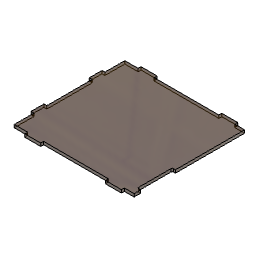
Deck Plate (Autodesk Fusion 360 design; units mm, degrees)
Autodesk Fusion 360 part; units mm, degrees
sketch "Sketch1" plane through (0, 0, 0) normal (0, 0, 1) x (1, 0, 0)
  line L0 (160, -90) -> (-160, -90)
  line L1 (-160, -90) -> (-160, 90)
  line L2 (-160, 90) -> (160, 90)
  line L3 (160, 90) -> (160, -90)
  line L4 (160, -90) -> (-160, 90) construction
  line L5 (-160, -90) -> (160, 90) construction
  line L6 (170, 85.5) -> (-180, 85.5) construction
  line L7 (-180, -85.5) -> (170, -85.5) construction
  line L8 (-155.5, 90) -> (-155.5, -90)
  line L9 (-160, 90) -> (-135, 90)
  line L10 (-135, 90) -> (-135, 85.5)
  line L11 (-135, 85.5) -> (-160, 85.5)
  line L12 (-160, 85.5) -> (-160, 90)
  line L13 (-160, -90) -> (-135, -90)
  line L14 (-135, -90) -> (-135, -85.5)
  line L15 (-135, -85.5) -> (-160, -85.5)
  line L16 (-160, -85.5) -> (-160, -90)
  line L17 (-110, -90) -> (-10, -90)
  line L18 (-10, -90) -> (-10, -85.5)
  line L19 (-10, -85.5) -> (-110, -85.5)
  line L20 (-110, -85.5) -> (-110, -90)
  line L21 (-10, -90) -> (15, -90)
  line L22 (15, -90) -> (15, -85.5)
  line L23 (15, -85.5) -> (-10, -85.5)
  line L24 (-10, -85.5) -> (-10, -90)
  line L25 (15, -90) -> (115, -90)
  line L26 (115, -85.5) -> (15, -85.5)
  line L27 (15, -85.5) -> (15, -90)
  line L28 (115, -90) -> (140, -90)
  line L29 (140, -85.5) -> (115, -85.5)
  line L30 (-135, 85.5) -> (-110, 85.5)
  line L31 (-110, 85.5) -> (-110, 90)
  line L32 (-110, 90) -> (-135, 90)
  line L33 (-135, 90) -> (-135, 85.5)
  line L34 (-110, 85.5) -> (-10, 85.5)
  line L35 (-10, 85.5) -> (-10, 90)
  line L36 (-10, 90) -> (-110, 90)
  line L37 (-110, 90) -> (-110, 85.5)
  line L38 (-10, 85.5) -> (15, 85.5)
  line L39 (15, 85.5) -> (15, 90)
  line L40 (15, 90) -> (-10, 90)
  line L41 (-10, 90) -> (-10, 85.5)
  line L42 (15, 85.5) -> (115, 85.5)
  line L43 (115, 90) -> (15, 90)
  line L44 (15, 90) -> (15, 85.5)
  line L45 (115, 85.5) -> (140, 85.5)
  line L46 (140, 90) -> (115, 90)
  line L47 (140, 85.5) -> (160, 85.5)
  line L48 (160, 85.5) -> (160, 90)
  line L49 (160, 90) -> (140, 90)
  line L50 (140, -90) -> (160, -90)
  line L51 (160, -90) -> (160, -85.5)
  line L52 (160, -85.5) -> (140, -85.5)
  line L53 (-160, 55) -> (-155.5, 55)
  line L54 (-155.5, 55) -> (-155.5, 35)
  line L55 (-155.5, 35) -> (-160, 35)
  line L56 (-160, 35) -> (-160, 55)
  line L57 (-160, -35) -> (-155.5, -35)
  line L58 (-155.5, -35) -> (-155.5, -55)
  line L59 (-155.5, -55) -> (-160, -55)
  line L60 (-160, -55) -> (-160, -35)
  line L61 (30, 90) -> (30, -90)
  line L62 (30, -75.5) -> (25, -75.5)
  line L63 (25, -75.5) -> (25, -21.5)
  line L64 (25, -21.5) -> (30, -21.5)
  line L65 (30, -21.5) -> (30, -75.5)
  point P0 (-15, -14)
  dimension "d1" = 320
  dimension "d2" = 180
  dimension "d3" = 4.5
  dimension "d4" = 4.5
  dimension "d5" = 4.5
  dimension "d6" = 25
  dimension "d7" = 25
  dimension "d8" = 100
  dimension "d9" = 25
  dimension "d10" = 25
  dimension "d13" = 25
  dimension "d14" = 100
  dimension "d15" = 25
  dimension "d18" = 20
  dimension "d19" = 20
  dimension "d20" = 35
  dimension "d21" = 35
  dimension "d46" = 15
  dimension "d55" = 5
  dimension "d56" = 54
  dimension "d58" = 10
  constraint horizontal L0
  constraint perpendicular L0 L1
  constraint parallel L0 L2
  constraint parallel L1 L3
  constraint coincident L4 origin
  constraint coincident L5 origin
  constraint perpendicular L3 L6
  constraint perpendicular L3 L7
  constraint perpendicular L0 L8
  constraint horizontal L9
  constraint vertical L10
  constraint horizontal L11
  constraint vertical L12
  constraint horizontal L13
  constraint vertical L14
  constraint horizontal L15
  constraint vertical L16
  constraint horizontal L17
  constraint vertical L18
  constraint horizontal L19
  constraint vertical L20
  constraint coincident L0 L17.start
  constraint horizontal L21
  constraint vertical L22
  constraint horizontal L23
  constraint vertical L24
  constraint horizontal L25
  constraint horizontal L26
  constraint vertical L27
  constraint horizontal L28
  constraint horizontal L29
  constraint horizontal L30
  constraint vertical L31
  constraint horizontal L32
  constraint vertical L33
  constraint horizontal L34
  constraint vertical L35
  constraint horizontal L36
  constraint vertical L37
  constraint horizontal L38
  constraint vertical L39
  constraint horizontal L40
  constraint vertical L41
  constraint horizontal L42
  constraint horizontal L43
  constraint vertical L44
  constraint horizontal L45
  constraint horizontal L46
  constraint horizontal L47
  constraint vertical L48
  constraint horizontal L49
  constraint horizontal L50
  constraint vertical L51
  constraint horizontal L52
  constraint coincident L3 L51.end
  constraint coincident L7 L51.end
  constraint horizontal L53
  constraint vertical L54
  constraint horizontal L55
  constraint vertical L56
  constraint coincident L1 L53.start
  constraint horizontal L57
  constraint vertical L58
  constraint horizontal L59
  constraint vertical L60
  constraint coincident L1 L57.start
  constraint coincident L2 L8.start
  constraint coincident L2 L61.start
  constraint coincident L43 L61.start
  constraint coincident L25 L61.end
  constraint perpendicular L25 L61
  constraint horizontal L62
  constraint vertical L63
  constraint horizontal L64
  constraint vertical L65
  constraint coincident L61 L62.start
  measures "d1" distance of L1.end L2.end
  measures "d2" distance of L0.end L1.end
  measures "d3" distance of L0 L7
  measures "d4" distance of L2 L6
  measures "d5" distance of L1 L8
  measures "d6" distance of L1.end L9.end
  measures "d7" distance of L0.end L13.end
  measures "d8" distance of L17.start L17.end
  measures "d9" distance of L14 L20
  measures "d10" distance of L17.end L21.end
  measures "d13" distance of L10.end L30.end
  measures "d14" distance of L30.end L34.end
  measures "d15" distance of L34.end L38.end
  measures "d18" distance of L53.start L55.end
  measures "d19" distance of L57.start L59.end
  measures "d20" distance of L13 L59
  measures "d21" distance of L9 L53
  measures "d46" distance of L39 L61
  measures "d55" distance of L62.start L62.end
  measures "d56" distance of L62.start L64.end
  measures "d58" distance of L7 L62
extrude "Extrude1" add sketch "Sketch1" along normal blind 4.5 contours L0 L18 L21 L22 L23 L24 L27 | L0 L8 L11 L14 L15 L19 L20 L23 L26 L30 L34 L38 L42 L54 L58 L61 L62 L63 L64 | L2 L35 L38 L39 L40 L41 L44 | L2 L10 L30 L31 L32 L33 L37 | L1 L8 L57 L58 L59 L60 | L1 L8 L53 L54 L55 L56
move_face "OffsetFaces1" offset -0.1 4 faces at (15, -88.5, 1.5) (-110, -87, 1.5) (-110, 87, 1.5) (15, 87, 1.5)
move_face "OffsetFaces2" offset -0.1 4 faces at (-10, -88.5, 1.5) (-135, -88.5, 3) (-10, 87, 1.5) (-135, 88.5, 1.5)
move_face "OffsetFaces3" offset -0.1 2 faces at (-158.5, -35, 1.5) (-158.5, 55, 1.5)
move_face "OffsetFaces4" offset -0.1 2 faces at (-157, -55, 1.5) (-157, 35, 1.5)
fillet "Fillet1" radius 2 2 edges at (25, -75.5, 2.25) (25, -21.5, 2.25)
